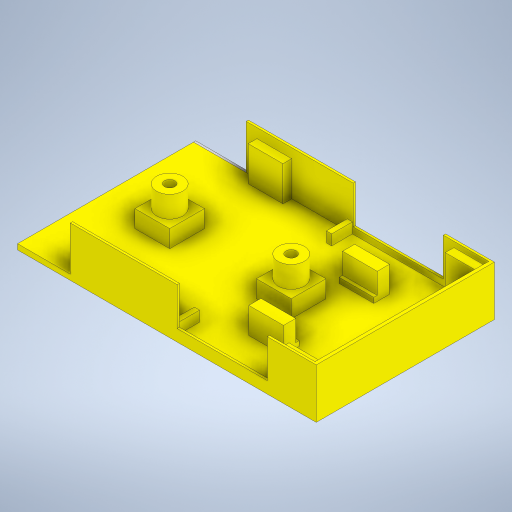
# Autodesk Inventor part: Sujeta_motor
Saved by Autodesk Inventor 2024 (Build 280153000, 153)
## iProperties
Created: 2024-04-23
Part Number: Sujeta_motor
Material: Generic
Document SubType Name: Modeling
Designer: samue
Density: 1 g/cm^3
Appearance: Default
Author: samue
## iProperties of the stored document Sujeta_motor_3DPrint.ipt
Created: 2024-05-02
Part Number: Sujeta_motor_3DPrint
Material: Generic
Document SubType Name: Modeling
Designer: samue
Density: 1 g/cm^3
Appearance: Default
Author: samue
Autodesk Inventor part; units mm, degrees
ref_plane "YZ Plane" through (0, 0, 0) normal (1, 0, 0) x (0, 1, 0)
ref_plane "XZ Plane" through (0, 0, 0) normal (0, 1, 0) x (-1, 0, 0)
ref_plane "XY Plane" through (0, 0, 0) normal (0, 0, 1) x (1, 0, 0)
sketch "Sketch1" plane through (0, 0, 0) normal (0, 1, 0) x (-1, 0, 0)
  line L0 (85, 50) -> (-85, 50)
  line L1 (-85, 50) -> (-85, -50)
  line L2 (-85, -50) -> (85, -50)
  line L3 (85, -50) -> (85, 50)
  line L4 (85, 50) -> (-85, -50) construction
  line L5 (-85, 50) -> (85, -50) construction
  point P0 (0, 0)
  dimension "d0" = 170
  dimension "d1" = 100
  constraints: 12 end point, 2 midpoint, 2 parallel, 1 horizontal, 1 perpendicular
  measures "d0" distance of L2.end L1.end
  measures "d1" distance of L1.end L0.end
extrude "Extrusion1" add sketch "Sketch1" along normal blind 3.125
sketch "Sketch2" plane through (0, 3.125, 0) normal (0, 1, 0) x (1, 0, 0)
  line L0 (-58.7056, 10) -> (-38.7056, 10)
  line L1 (-38.7056, 10) -> (-38.7056, -10)
  line L2 (-38.7056, -10) -> (-58.7056, -10)
  line L3 (-58.7056, -10) -> (-58.7056, 10)
  line L4 (-58.7056, 10) -> (-38.7056, -10) construction
  line L5 (-38.7056, 10) -> (-58.7056, -10) construction
  circle A0 centre (-48.7056, 0) radius 7.5
  line L6 (11.271, 10) -> (31.271, 10)
  line L7 (31.271, 10) -> (31.271, -10)
  line L8 (31.271, -10) -> (11.271, -10)
  line L9 (11.271, -10) -> (11.271, 10)
  line L10 (11.271, 10) -> (31.271, -10) construction
  line L11 (31.271, 10) -> (11.271, -10) construction
  circle A1 centre (21.271, 0) radius 7.5
  point P0 (0, 0)
  dimension "d4" = 20
  dimension "d5" = 20
  dimension "d6" = 15
  dimension "d14" = 20
  dimension "d15" = 20
  dimension "d16" = 15
  constraints: 24 end point, 4 midpoint, 4 parallel, 2 centre point, 2 coincident, 2 horizontal, 2 perpendicular, 1 horizontal alignment
  measures "d4" distance of L1.end L2.end
  measures "d5" distance of L0.end L1.end
  measures "d6" diameter of A0
  measures "d14" distance of L7.end L8.end
  measures "d15" distance of L6.end L7.end
  measures "d16" diameter of A1
extrude "Extrusion2" add sketch "Sketch2" along normal blind 22.4 contours A0 | A1
extrude "Extrusion3" add sketch "Sketch2" along normal blind 10 contours L0 L1 L2 L3 | L6 L7 L8 L9 | A1
sketch "Sketch3" plane through (-48.7056, 25.525, 0) normal (0, 1, 0) x (1, 0, 0)
  circle A0 centre (0, 0) radius 3
  point P0 (48.7056, 0)
  dimension "d11" = 6
  constraints: 1 centre point
  measures "d11" diameter of A0
extrude "Extrusion4" cut sketch "Sketch3" against normal blind 7
sketch "Sketch4" plane through (21.271, 25.525, 0) normal (0, 1, 0) x (1, 0, 0)
  circle A0 centre (0, 0) radius 3
  point P0 (-21.271, 0)
  dimension "d17" = 6
  constraints: 1 centre point
  measures "d17" diameter of A0
extrude "Extrusion5" cut sketch "Sketch4" against normal blind 7
sketch "Sketch5" plane through (0, 3.125, 0) normal (0, 1, 0) x (1, 0, 0)
  line L0 (85, 50) -> (-85, 50) projected
  line L1 (-85, 50) -> (85, 50)
  line L2 (85, 50) -> (85, 51.3)
  line L3 (85, 51.3) -> (-85, 51.3)
  line L4 (-85, 51.3) -> (-85, 50)
  line L5 (-85, -50) -> (85, -50) projected
  line L6 (-85, -50) -> (85, -50)
  line L7 (85, -50) -> (85, -51.3)
  line L8 (85, -51.3) -> (-85, -51.3)
  line L9 (-85, -51.3) -> (-85, -50)
  line L10 (85, -51.3) -> (87, -51.3)
  line L11 (87, -51.3) -> (87, 51.3)
  line L12 (87, 51.3) -> (85, 51.3)
  line L13 (85, 51.3) -> (85, -51.3)
  point P0 (0, 0)
  point P1 (85, -50)
  dimension "d20" = 1.3
  dimension "d21" = 1.3
  dimension "d22" = 2
  constraints: 24 end point, 6 parallel, 3 horizontal, 3 perpendicular
  measures "d20" distance of L2.end L1.end
  measures "d21" distance of L6.end L7.end
  measures "d22" distance of L12.end L11.end
extrude "Extrusion6" add sketch "Sketch5" along normal blind 25.525
sketch "Sketch6" plane through (-85, 0, 50) normal (0, 0, 1) x (1, 0, 0)
  line L0 (170, 0) -> (0, 0) projected
  line L1 (170, 0) -> (170, 3.125) projected
  line L2 (0, 0) -> (170, 0)
  line L3 (170, 0) -> (170, 3.125)
  line L4 (170, 3.125) -> (0, 3.125)
  line L5 (0, 3.125) -> (0, 0)
  point P0 (85, 0)
  constraints: 8 end point, 2 parallel, 1 horizontal, 1 perpendicular
extrude "Extrusion7" add sketch "Sketch6" along normal blind 1.3
sketch "Sketch7" plane through (85, 0, -50) normal (0, 0, -1) x (-1, 0, 0)
  line L0 (0, 0) -> (0, 3.125) projected
  line L1 (170, 0) -> (170, 28.65) projected
  line L2 (0, 0) -> (170, 0)
  line L3 (170, 0) -> (170, 2.2028)
  line L4 (170, 2.2028) -> (0, 2.2028)
  line L5 (0, 2.2028) -> (0, 0)
  constraints: 8 end point, 2 parallel, 1 horizontal, 1 perpendicular, 1 point on line
extrude "Extrusion8" add sketch "Sketch7" along normal blind 1.3
sketch "Sketch8" plane through (85, 0, 51.3) normal (1, 0, 0) x (0, 0, -1)
  line L0 (0, 0) -> (0, 3.125) projected
  line L1 (0, 0) -> (102.6, 0) projected
  line L2 (0, 3.125) -> (102.6, 3.125)
  line L3 (102.6, 3.125) -> (102.6, 0)
  line L4 (102.6, 0) -> (0, 0)
  line L5 (0, 0) -> (0, 3.125)
  point P0 (51.3, 0)
  constraints: 8 end point, 2 parallel, 1 horizontal, 1 perpendicular
extrude "Extrusion9" add sketch "Sketch8" along normal blind 2
sketch "Sketch9" plane through (0, 3.125, 0) normal (0, 1, 0) x (1, 0, 0)
  line L0 (85, -50) -> (85, 50) projected
  line L1 (85, 50) -> (65, 50)
  line L2 (65, 50) -> (65, 45)
  line L3 (65, 45) -> (85, 45)
  line L4 (85, 45) -> (85, 50)
  line L5 (85, -50) -> (65, -50)
  line L6 (65, -50) -> (65, -45)
  line L7 (65, -45) -> (85, -45)
  line L8 (85, -45) -> (85, -50)
  point P0 (0, 0)
  dimension "d31" = 20
  dimension "d32" = 5
  dimension "d33" = 20
  dimension "d34" = 5
  constraints: 16 end point, 4 parallel, 2 horizontal, 2 perpendicular
  measures "d31" distance of L3.end L2.end
  measures "d32" distance of L2.end L1.end
  measures "d33" distance of L6.end L7.end
  measures "d34" distance of L5.end L6.end
extrude "Extrusion10" add sketch "Sketch9" along normal blind 22.4
sketch "Sketch10" plane through (-85, 3.125, 50) normal (0, 0, -1) x (-1, 0, 0)
  line L0 (-170, 25.525) -> (0, 25.525) projected
  line L1 (-143.8389, 3.6428) -> (-91.9175, 3.6428)
  line L2 (-91.9175, 3.6428) -> (-91.9175, 25.525)
  line L3 (-91.9175, 25.525) -> (-143.8389, 25.525)
  line L4 (-143.8389, 25.525) -> (-143.8389, 3.6428)
  point P0 (-150, 27.4)
  point P1 (-143.8389, 25.525)
  constraints: 8 end point, 2 parallel, 1 horizontal, 1 perpendicular, 2 other
extrude "Extrusion11" cut sketch "Sketch10" against normal blind 27.4
mirror "Mirror1" about plane through (0, 0, 0) normal (0, 0, 1) of "Extrusion11"
sketch "Sketch11" plane through (0, 3.125, 0) normal (0, 1, 0) x (1, 0, 0)
  line L0 (47.3531, -30.5) -> (27.3531, -30.5)
  line L1 (27.3531, -30.5) -> (27.3531, -23.5)
  line L2 (27.3531, -23.5) -> (47.3531, -23.5)
  line L3 (47.3531, -23.5) -> (47.3531, -30.5)
  line L4 (-85, -50) -> (65, -50) projected
  point P0 (0, 0)
  dimension "d39" = 7
  dimension "d42" = 19.5
  dimension "d43" = 20
  constraints: 8 end point, 2 parallel, 1 horizontal, 1 perpendicular
  measures "d39" distance of L0.end L1.end
  measures "d42" distance between parallel lines of L0 L4
  measures "d43" distance of L1.end L2.end
extrude "Extrusion12" add sketch "Sketch11" along normal blind 15
sketch "Sketch12" plane through (0, 3.125, 0) normal (0, 1, 0) x (1, 0, 0)
  line L0 (27.3531, -23.5) -> (47.3531, -23.5) projected
  line L1 (47.3531, -23.5) -> (27.3531, -23.5)
  line L2 (27.3531, -23.5) -> (27.3531, -21.5)
  line L3 (27.3531, -21.5) -> (47.3531, -21.5)
  line L4 (47.3531, -21.5) -> (47.3531, -23.5)
  point P0 (0, 0)
  dimension "d44" = 2
  constraints: 8 end point, 2 parallel, 1 horizontal, 1 perpendicular
  measures "d44" distance of L1.end L2.end
extrude "Extrusion13" add sketch "Sketch12" along normal blind 3
mirror "Mirror2" about plane through (0, 0, 0) normal (0, 0, 1) of "Extrusion12", "Extrusion13"
sketch "Sketch13" plane through (0, 3.125, 0) normal (0, 1, 0) x (1, 0, 0)
  line L0 (-85, -50) -> (65, -50) projected
  line L1 (6.5534, -50) -> (3.5534, -50)
  line L2 (3.5534, -50) -> (3.5534, -38)
  line L3 (3.5534, -38) -> (6.5534, -38)
  line L4 (6.5534, -38) -> (6.5534, -50)
  point P0 (0, 0)
  dimension "d47" = 3
  dimension "d48" = 12
  constraints: 8 end point, 2 parallel, 1 horizontal, 1 perpendicular, 1 point on line
  measures "d47" distance of L2.end L3.end
  measures "d48" distance of L1.end L2.end
extrude "Extrusion14" add sketch "Sketch13" along normal blind 6
mirror "Mirror3" about plane through (0, 0, 0) normal (0, 0, 1) of "Extrusion14"
sketch "Sketch14" plane through (0, 3.125, 0) normal (0, 1, 0) x (1, 0, 0)
  line L0 (-85, -50) -> (3.5534, -50) projected
  line L1 (-28.4579, -50) -> (-48.4579, -50)
  line L2 (-48.4579, -50) -> (-48.4579, -45)
  line L3 (-48.4579, -45) -> (-28.4579, -45)
  line L4 (-28.4579, -45) -> (-28.4579, -50)
  point P0 (0, 0)
  dimension "d51" = 20
  dimension "d52" = 5
  constraints: 8 end point, 2 parallel, 1 horizontal, 1 perpendicular, 1 point on line
  measures "d51" distance of L2.end L3.end
  measures "d52" distance of L1.end L2.end
extrude "Extrusion15" add sketch "Sketch14" along normal blind 20
mirror "Mirror4" about plane through (0, 0, 0) normal (0, 0, 1) of "Extrusion15"
sketch "Sketch15" plane through (-85, 3.125, 50) normal (0, 0, -1) x (-1, 0, 0)
  line L0 (0, 0) -> (-36.5421, 0) projected
  line L1 (-91.9175, 25.525) -> (0, 25.525) projected
  line L2 (0, 0) -> (-30.3469, 0)
  line L3 (-30.3469, 0) -> (-30.3469, 25.525)
  line L4 (-30.3469, 25.525) -> (0, 25.525)
  line L5 (0, 25.525) -> (0, 0)
  point P0 (-85, -3.125)
  point P1 (0, 25.525)
  point P2 (-30.3469, 0)
  constraints: 8 end point, 2 parallel, 1 horizontal, 1 perpendicular, 1 point on line
extrude "Extrusion16" cut sketch "Sketch15" against normal blind 20
mirror "Mirror5" about plane through (0, 0, 0) normal (0, 0, 1) of "Extrusion16"
sketch "Sketch17" plane through (-85, 2.2028, -50) normal (0, 1, 0) x (1, 0, 0)
  line L0 (170, 0) -> (0, 0) projected
  line L1 (0, 0) -> (170, 0)
  line L2 (170, 0) -> (170, 1.3)
  line L3 (170, 1.3) -> (0, 1.3)
  line L4 (0, 1.3) -> (0, 0)
  point P0 (85, -50)
  constraints: 8 end point, 2 parallel, 1 horizontal, 1 perpendicular
extrude "Extrusion19" add sketch "Sketch17" along normal blind 0.922
body "Solid1"
